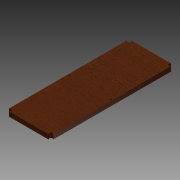
# Autodesk Inventor part: Mid
Saved by Autodesk Inventor 2015 (Build 190159000, 159)
## iProperties
Created: 2014-07-25
Part Number: Mid
Material: Wood (Walnut)
Document SubType Name: Modeling
Designer: Michael
Density: 0.55 g/cm^3
Appearance: Walnut - Natural Polished
Author: Michael
Autodesk Inventor part; units mm, degrees
ref_plane "YZ Plane" through (0, 0, 0) normal (1, 0, 0) x (0, 1, 0)
ref_plane "XZ Plane" through (0, 0, 0) normal (0, 1, 0) x (-1, 0, 0)
ref_plane "XY Plane" through (0, 0, 0) normal (0, 0, 1) x (1, 0, 0)
sketch "Sketch1" plane through (0, 0, 0) normal (0, 1, 0) x (-1, 0, 0)
  line L0 (-0.444009, 225.316004) -> (-86.169009, 225.316004)
  line L1 (-89.344009, 222.141004) -> (-89.344009, -25.508996)
  line L2 (-86.169009, -28.683996) -> (-0.444009, -28.683996)
  line L3 (2.730991, -25.508996) -> (2.730991, 222.141004)
  arc A0 (-86.169009, -28.683996) -> (-89.344009, -25.508996) centre (-86.169009, -25.508996) ccw
  arc A1 (-0.444009, 225.316004) -> (2.730991, 222.141004) centre (-0.444009, 222.141004) ccw
  arc A2 (-89.344009, 222.141004) -> (-86.169009, 225.316004) centre (-86.169009, 222.141004) ccw
  arc A3 (2.730991, -25.508996) -> (-0.444009, -28.683996) centre (-0.444009, -25.508996) ccw
  circle A4 centre (-0.444009, 98.316004) radius 1.4732
  circle A5 centre (-86.169009, 98.316004) radius 1.4732
  point P0 (0, 0)
  dimension "d2" = 6.35
  dimension "d3" = 6.35
  dimension "d4" = 6.35
  dimension "d5" = 6.35
  dimension "d7" = 2.9464
  dimension "d8" = 2.9464
  constraints: 8 end point, 8 point on circle, 6 centre point
  measures "d2" diameter of A0
  measures "d3" diameter of A1
  measures "d4" diameter of A2
  measures "d5" diameter of A3
  measures "d7" diameter of A4
  measures "d8" diameter of A5
sketch "Sketch1 outline for Extrusion1" plane through (0, 0, 0) normal (0, 1, 0) x (-1, 0, 0)
  arc A0 (2.730991, 222.141004) -> (-0.444009, 225.316004) centre (-0.444009, 222.141004) cw
  line L0 (2.730991, -25.508996) -> (2.730991, 222.141004)
  line L1 (-0.444009, 225.316004) -> (-86.169009, 225.316004)
  arc A1 (-0.444009, -28.683996) -> (2.730991, -25.508996) centre (-0.444009, -25.508996) cw
  arc A2 (-86.169009, 225.316004) -> (-89.344009, 222.141004) centre (-86.169009, 222.141004) cw
  line L2 (-86.169009, -28.683996) -> (-0.444009, -28.683996)
  line L3 (-89.344009, 222.141004) -> (-89.344009, -25.508996)
  arc A3 (-89.344009, -25.508996) -> (-86.169009, -28.683996) centre (-86.169009, -25.508996) cw
  circle A4 centre (-86.169009, 98.316004) radius 1.4732
  circle A5 centre (-0.444009, 98.316004) radius 1.4732
extrude "Extrusion1" add sketch "Sketch1 outline for Extrusion1" along normal blind 9.525
fillet "Fillet1" radius 0.3175 8 edges at (86.169, 4.7625, 225.316) (89.344, 4.7625, 222.141) (0.444, 4.7625, 225.316) (-2.731, 4.7625, 222.141) (-2.731, 4.7625, -25.509) (0.444, 4.7625, -28.684) (86.169, 4.7625, -28.684) (89.344, 4.7625, -25.509)
body "Solid1"
